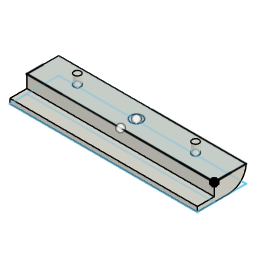
fumehood-glass-holder (Autodesk Fusion 360 design; units mm, degrees)
Autodesk Fusion 360 part; units mm, degrees
sketch "Sketch1" plane through (0, 0, 0) normal (0, 0, 1) x (1, 0, 0)
  line L0 (-7.5, 2.5) -> (46.7, 2.5)
  line L1 (46.7, 2.5) -> (46.7, -11.6)
  line L2 (46.7, -11.6) -> (-7.5, -11.6)
  line L3 (-7.5, -11.6) -> (-7.5, 2.5)
  line L4 (46.7, -11.6) -> (-7.5, -11.6)
  line L5 (-7.5, -11.6) -> (-7.5, -6.7)
  line L6 (-7.5, -6.7) -> (46.7, -6.7)
  line L7 (46.7, -6.7) -> (46.7, -11.6)
  dimension "d1" = 54.2
  dimension "d2" = 14.1
  dimension "d3" = 4.9
  constraint horizontal L0
  constraint vertical L1
  constraint horizontal L2
  constraint vertical L3
  constraint horizontal L4
  constraint vertical L5
  constraint horizontal L6
  constraint vertical L7
  constraint coincident L3 L5.end
  measures "d1" distance of L0.start L0.end
  measures "d2" distance of L0.start L2.end
  measures "d3" distance of L1.end L6.end
extrude "Extrude1" add sketch "Sketch1" along normal blind 5 contours L0 L1 L3 L6
extrude "Extrude2" add sketch "Sketch1" along normal blind 1.35 contours L1 L2 L3 L4 L5 L6 L7
sketch "Sketch2" plane through (0, 0, 5) normal (0, 0, 1) x (-1, 0, 0)
  line L0 (7.5, -2.5) -> (7.5, 6.7)
  line L1 (7.5, 6.7) -> (-46.7, 6.7)
  line L2 (-46.7, 6.7) -> (-46.7, -2.5)
  line L3 (-46.7, -2.5) -> (7.5, -2.5)
  line L4 (-19.6, -2.5) -> (-46.7, -2.5)
  line L5 (-46.7, -2.5) -> (-46.7, 6.7)
  line L6 (-46.7, 6.7) -> (-19.6, 6.7)
  line L7 (-46.7, 2.1) -> (-46.7, 6.7)
  line L8 (-46.7, 6.7) -> (7.5, 6.7)
  line L9 (7.5, 6.7) -> (7.5, 2.1)
  circle A0 centre (-19.6, 2.1) radius 1.7
  line L10 (-36.7, 6.7) -> (-46.7, 6.7)
  line L11 (-46.7, 6.7) -> (-46.7, 2.1)
  line L12 (-2.5, 6.7) -> (7.5, 6.7)
  line L13 (7.5, 6.7) -> (7.5, 2.1)
  circle A1 centre (-2.5, 2.1) radius 1
  circle A2 centre (-36.7, 2.1) radius 1
  dimension "d8" = 3.4
  dimension "d9" = 10
  dimension "d10" = 10
  dimension "d11" = 2
  dimension "d12" = 2
  constraint horizontal L4
  constraint vertical L5
  constraint horizontal L6
  constraint coincident L1.end L2.start
  constraint midpoint L3 L4.start
  constraint vertical L7
  constraint horizontal L8
  constraint vertical L9
  constraint midpoint L0 L9.end
  constraint horizontal L10
  constraint vertical L11
  constraint coincident L6 L10.start
  constraint horizontal L12
  constraint vertical L13
  constraint coincident L8 L12.start
  measures "d8" diameter of A0
  measures "d9" distance of L7.start A2.centre
  measures "d10" distance of L9.end A1.centre
  measures "d11" diameter of A1
  measures "d12" diameter of A2
extrude "Extrude3" cut sketch "Sketch2" against normal blind 18 contours A0
extrude "Extrude4" add sketch "Sketch2" along normal blind 2.9 contours A1 | A2
sketch "Sketch3" plane through (-7.5, 0, 0) normal (-1, 0, 0) x (0, -1, 0)
  line L0 (-2.5, 0) -> (11.6, 0)
  line L1 (11.6, 0) -> (11.6, 1.35)
  line L2 (11.6, 1.35) -> (6.7, 1.35)
  line L3 (6.7, 1.35) -> (6.7, 5)
  line L4 (6.7, 5) -> (-2.5, 5)
  line L5 (-2.5, 5) -> (-2.5, 0)
  line L6 (-2.5, 5) -> (2.5, 5)
  line L7 (2.5, 5) -> (2.5, 0)
  line L8 (2.5, 0) -> (-2.5, 0)
  line L9 (-2.5, 0) -> (-2.5, 5)
  circle A0 centre (2.5, 5) radius 5
  dimension "d17" = 5
  constraint horizontal L6
  constraint vertical L7
  constraint horizontal L8
  constraint vertical L9
  constraint coincident L0 L7.end
  constraint coincident L4.end L5.start
  constraint coincident L6.end L7.start
  constraint coincident L4.end A0
  measures "d17" distance of L4.end L6.end
extrude "Extrude5" cut sketch "Sketch3" against normal blind 63 contours L0 L5 L8 L9 A0
